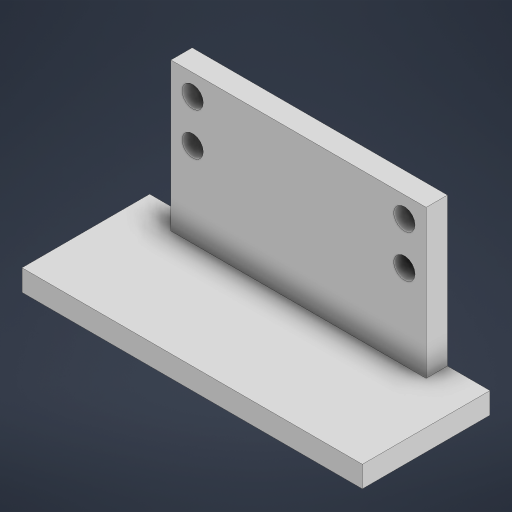
# Autodesk Inventor part: fp v2 servo Mounting
Saved by Autodesk Inventor 2023.6 (Build 276521000, 521)
## iProperties
Created: 2026-02-24
Part Number: fp v2 servo Mounting
Material: Generic
Document SubType Name: Modeling
Designer: user
Density: 1 g/cm^3
Appearance: Default
Author: user
Autodesk Inventor part; units mm, degrees
ref_plane "YZ Plane" through (0, 0, 0) normal (1, 0, 0) x (0, 1, 0)
ref_plane "XZ Plane" through (0, 0, 0) normal (0, 1, 0) x (-1, 0, 0)
ref_plane "XY Plane" through (0, 0, 0) normal (0, 0, 1) x (1, 0, 0)
sketch "Sketch1" plane through (0, 0, 0) normal (0, 0, 1) x (1, 0, 0)
  line L0 (-30, 19.8) -> (30, 19.8)
  line L1 (30, 19.8) -> (30, 0)
  line L2 (30, 0) -> (-30, 0)
  line L3 (-30, 0) -> (-30, 19.8)
  line L4 (-30, 0) -> (30, 0)
  line L5 (30, 0) -> (30, -15)
  line L6 (30, -15) -> (-30, -15)
  line L7 (-30, -15) -> (-30, 0)
  line L8 (-30, -15) -> (30, -15)
  line L9 (30, -15) -> (30, -20)
  line L10 (30, -20) -> (-30, -20)
  line L11 (-30, -20) -> (-30, -15)
  line L12 (-30, -17.5) -> (30, -17.5)
  line L13 (-40, -15) -> (40, -15)
  line L14 (40, -15) -> (40, -20)
  line L15 (40, -20) -> (-40, -20)
  line L16 (-40, -20) -> (-40, -15)
  line L17 (-40, -15) -> (40, -20) construction
  line L18 (40, -15) -> (-40, -20) construction
  line L19 (0, 0) -> (0, -20)
  point P0 (0, -17.5)
  point P1 (-40, -17.5)
  point P2 (-30, -15)
  dimension "d0" = 60
  dimension "d1" = 19.8
  dimension "d2" = 15
  dimension "d5" = 5
  dimension "d6" = 80
  constraints: 40 end point, 8 midpoint, 8 parallel, 4 horizontal, 4 perpendicular, 1 coincident, 1 point on line
  measures "d0" distance between parallel lines of L1 L3
  measures "d1" distance between parallel lines of L2 L0
  measures "d2" distance between parallel lines of L6 L2
  measures "d5" distance between parallel lines of L10 L6
  measures "d6" distance from line of L14 point (-40, -17.5)
extrude "Extrusion1" add sketch "Sketch1" along normal blind 5 contours L0 L1 L2 L3 | L2 L19 L6 L7 | L5 L6 L19 L2
extrude "Extrusion2" add sketch "Sketch1" along normal blind 30 contours L6 L19 L12 L11 | L11 L15 L16 L13 | L9 L12 L19 L6 | L13 L14 L15 L9 | L12 L19 L10 L11 | L9 L10 L19 L12
sketch "Sketch2" plane through (0, 0, 5) normal (0, 0, 1) x (1, 0, 0)
  line L0 (-30, -15) -> (30, -15) projected
  line L1 (-29.9232, 0) -> (30, 0)
  line L2 (30, 0) -> (30, -15)
  line L3 (30, -15) -> (-29.9232, -15)
  line L4 (-29.9232, -15) -> (-29.9232, 0)
  line L5 (-30, 19.8) -> (-30, -15) projected
  line L6 (-30, 4.9) -> (30.0951, 4.9)
  line L7 (-30, 14.9) -> (30, 14.9)
  line L8 (30, -15) -> (30, 19.8) projected
  line L9 (30, 19.8) -> (-30, 19.8) projected
  circle A0 centre (-24.89, 4.9) radius 2.5
  circle A1 centre (24.89, 4.9) radius 2.5
  line L10 (-24.89, 4.9) -> (24.89, 4.9)
  line L11 (0, 0) -> (0, 4.9)
  line L12 (-30, 14.9) -> (-30, 4.9)
  line L13 (-30, 9.9) -> (30, 9.9)
  circle A2 centre (-24.89, 14.9) radius 2.5
  circle A3 centre (24.89, 14.9) radius 2.5
  dimension "d9" = 15
  dimension "d10" = 4.9
  dimension "d11" = 4.9
  dimension "d12" = 5
  dimension "d13" = 5
  dimension "d14" = 49.78
  dimension "d15" = 24.89
  constraints: 20 end point, 6 point on line, 4 centre point, 3 horizontal, 3 perpendicular, 2 collinear, 2 midpoint, 2 parallel, 2 symmetric about line, 2 other
  measures "d9" distance between parallel lines of L0 L1
  measures "d10" distance between parallel lines of L1 L6
  measures "d11" distance between parallel lines of L9 L7
  measures "d12" diameter of A0
  measures "d13" diameter of A1
  measures "d14" distance of L10.end L10.start
  measures "d15" distance from line of L10.end L11
extrude "Extrusion3" cut sketch "Sketch2" against normal blind 30 contours A0 L6 | L6 A0 | A2 L7 | L7 A2 | A1 L6 | L6 A1 | A3 L7 | L7 A3
body "Solid1"
